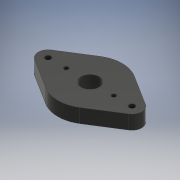
# Autodesk Inventor part: AC07
Saved by Autodesk Inventor 2017 (Build 210142000, 142)
## iProperties
Created: 2019-09-30
Part Number: AC07
Material: ABS Plastic
Document SubType Name: Modeling
Designer: Dell
Density: 1.06 g/cm^3
Appearance: Smooth - Black
Author: Dell
Autodesk Inventor part; units mm, degrees
ref_plane "YZ Plane" through (0, 0, 0) normal (1, 0, 0) x (0, 1, 0)
ref_plane "XZ Plane" through (0, 0, 0) normal (0, 1, 0) x (-1, 0, 0)
ref_plane "XY Plane" through (0, 0, 0) normal (0, 0, 1) x (1, 0, 0)
sketch "Sketch1" plane through (0, 0, 0) normal (0, 0, 1) x (1, 0, 0)
  circle A0 centre (0, 0) radius 11.5
  circle A1 centre (0, 0) radius 3.25
  circle A2 centre (8.5, 0) radius 0.75
  circle A3 centre (-8.5, 0) radius 0.75
  dimension "d0" = 23
  dimension "d1" = 6.5
  dimension "d2" = 1.5
  dimension "d3" = 8.5
  dimension "d6" = 360
  constraints: 4 centre point, 2 coincident, 1 horizontal alignment, 5 other
  measures "d0" diameter of A0
  measures "d1" diameter of A1
  measures "d2" diameter of A2
  measures "d3" distance of point (0, 0) A2.centre
extrude "Extrusion1" add sketch "Sketch1" along normal blind 5
sketch "Sketch3" plane through (0, 0, 5) normal (0, 0, 1) x (1, 0, 0)
  circle A0 centre (15, 0) radius 1
  circle A1 centre (15, 0) radius 3.5
  circle A2 centre (0, 0) radius 11.5 projected
  line L0 (6.1333, 9.7279) -> (16.8667, 2.9607)
  line L1 (16.8667, -2.9607) -> (6.1333, -9.7279)
  circle A3 centre (0, 0) radius 11.5 projected
  arc A4 (6.1333, -9.7279) -> (6.1333, 9.7279) centre (0, 0) ccw
  circle A5 centre (-15, 0) radius 1
  circle A6 centre (-15, 0) radius 3.5
  line L2 (-6.1333, -9.7279) -> (-16.8667, -2.9607)
  line L3 (-16.8667, 2.9607) -> (-6.1333, 9.7279)
  arc A7 (-6.1333, 9.7279) -> (-6.1333, -9.7279) centre (0, 0) ccw
  dimension "d17" = 2
  dimension "d18" = 15
  dimension "d21" = 360
  constraints: 10 point on circle, 8 end point, 7 tangent, 6 centre point, 2 coincident, 1 horizontal alignment, 25 other
  measures "d17" diameter of A0
  measures "d18" distance of A0.centre point (0, 0)
extrude "Extrusion3" add sketch "Sketch3" against normal blind 5 contours A1 | A1 A2 L0 | L1 A2 A1 | A2 A6 L3 | L2 A6 A2 | A6
body "Solid1"
